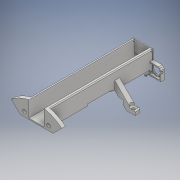
# Autodesk Inventor part: Hull_batt_pillar2
Saved by Autodesk Inventor 2018 (Build 220112000, 112)
## iProperties
Created: 2018-05-01
Part Number: Hull_batt_pillar2
Material: Generic
Document SubType Name: Modeling
Designer: suchanek
Density: 1 g/cm^3
Appearance: Default
Author: suchanek
Autodesk Inventor part; units mm, degrees
ref_plane "YZ Plane" through (0, 0, 0) normal (1, 0, 0) x (0, 1, 0)
ref_plane "XZ Plane" through (0, 0, 0) normal (0, 1, 0) x (-1, 0, 0)
ref_plane "XY Plane" through (0, 0, 0) normal (0, 0, 1) x (1, 0, 0)
sketch "Sketch1" plane through (0, 0, 0) normal (0, 1, 0) x (-1, 0, 0)
  arc A0 (21.0006, 25.4554) -> (6.35, 32.3833) centre (0, 0) ccw
  line L0 (0, 0) -> (-23.3345, 23.3345)
  line L1 (0, 0) -> (33, 0) construction
  line L2 (0, 0) -> (0, 8.3369)
  line L3 (-23.3345, 23.3345) -> (-9.1924, 9.1924)
  line L4 (-9.1924, 9.1924) -> (-6.965, 11.4198)
  line L5 (-6.965, 11.4198) -> (-13.7089, 18.1636)
  line L6 (-21.1071, 25.5619) -> (-23.3345, 23.3345)
  line L7 (23.3345, 23.3345) -> (9.1924, 9.1924)
  line L8 (9.1924, 9.1924) -> (6.965, 11.4198)
  line L9 (6.965, 11.4198) -> (13.7089, 18.1636)
  line L10 (21.1071, 25.5619) -> (23.3345, 23.3345)
  line L11 (-6.35, 32.3833) -> (6.35, 32.3833)
  line L12 (6.35, 32.3833) -> (6.35, 19.1636)
  line L13 (6.35, 19.1636) -> (-6.35, 19.1636)
  line L14 (-6.35, 19.1636) -> (-6.35, 32.3833)
  line L15 (13.7089, 18.1636) -> (-13.7089, 18.1636)
  line L16 (-13.7089, 18.1636) -> (-21.1071, 25.5619)
  arc A1 (-6.35, 32.3833) -> (-21.0006, 25.4554) centre (0, 0) ccw
  arc A2 (6.35, 32.3833) -> (-6.35, 32.3833) centre (0, 0) ccw
  line L17 (13.7089, 18.1636) -> (21.1071, 25.5619)
  point P0 (-6.35, 31.3636)
  dimension "d0" = 33
  dimension "d1" = 33
  dimension "d2" = 135
  dimension "d3" = 3.15
  dimension "d4" = 20
  dimension "d5" = 32
  dimension "d7" = 12.2
  dimension "d8" = 12.7
  dimension "d33" = 18.1636
  constraints: 36 end point, 7 point on circle, 6 point on line, 5 parallel, 4 symmetric about line, 3 centre point, 3 horizontal, 2 perpendicular, 1 coincident, 1 equal length, 1 vertical
  measures "d0" radius of A0
  measures "d1" distance of L0.start L0.end
  measures "d2" angle of L1 L0
  measures "d3" distance of L4.end L3.end
  measures "d4" distance between parallel lines of L6 L4
  measures "d5" distance of point (0, 0) point (-6.35, 31.364)
  measures "d7" distance of L13.end point (-6.35, 31.364)
  measures "d8" distance of L12.end L13.end
  measures "d33" distance from line of L0.start L15
extrude "Extrusion1" add sketch "Sketch1" along normal blind 3 contours L17 L15 L16 A1 L14 L13 L12 A0
sketch "Sketch2" plane through (0, 3, 0) normal (0, 1, 0) x (1, 0, 0)
  arc A0 (6.35, -32.3833) -> (21.0006, -25.4554) centre (0, 0) ccw projected
  line L0 (8.35, -31.9261) -> (8.35, -18.1636)
  line L1 (13.7089, -18.1636) -> (-13.7089, -18.1636) projected
  line L2 (-8.35, -18.1636) -> (-8.35, -31.9261)
  arc A1 (-21.0006, -25.4554) -> (-6.35, -32.3833) centre (0, 0) ccw projected
  line L3 (-6.35, -19.1636) -> (6.35, -19.1636) projected
  line L4 (6.35, -32.3833) -> (6.35, -19.1636)
  line L5 (6.35, -19.1636) -> (-6.35, -19.1636)
  line L6 (-6.35, -32.3833) -> (-6.35, -19.1636) projected
  line L7 (-6.35, -19.1636) -> (-6.35, -32.3833)
  dimension "d14" = 2
  constraints: 10 end point, 3 vertical, 2 perpendicular, 2 point on circle, 2 point on line, 1 horizontal alignment
  measures "d14" distance between parallel lines of L6 L2
extrude "Extrusion2" add sketch "Sketch2" along normal blind 85
ref_plane "Work Plane1" through (8.35, 3, 18.1636) normal (-0.7071068, 0, -0.7071068) x (0, 1, 0)
sketch "Sketch4" plane through (8.35, 3, 18.1636) normal (-0.7071068, 0, -0.7071068) x (0, 1, 0)
  circle A0 centre (49, 6.9393) radius 8
  line L0 (85, -9.7316) -> (85, 0) projected
  line L1 (-3, 3.7893) -> (0, 3.7893) projected
  line L2 (49, -1.0607) -> (31, -1.0607)
  line L3 (31, -1.0607) -> (31, 14.9393)
  line L4 (31, 14.9393) -> (49, 14.9393)
  line L5 (49, 14.9393) -> (49, -1.0607)
  point P0 (-3, 6.9393)
  dimension "d19" = 16
  dimension "d20" = 36
  dimension "d21" = 3.15
  dimension "d22" = 18
  dimension "d23" = 16
  constraints: 8 end point, 2 parallel, 2 point on circle, 1 centre point, 1 horizontal, 1 perpendicular
  measures "d19" diameter of A0
  measures "d20" distance from line of L0 A0.centre
  measures "d21" distance from line of L1 A0.centre
  measures "d22" distance of L3.end L4.end
  measures "d23" distance of L2.end L3.end
extrude "Extrusion3" cut sketch "Sketch4" along normal through all both and the other way through all
ref_plane "Work Plane3" through (0, 88, 18.1636) normal (-1, 0, 0) x (0, 0, 1)
mirror "Mirror1" about plane through (0, 88, 18.1636) normal (-1, 0, 0) of "Extrusion3"
sketch "Sketch5" plane through (0, 88, 0) normal (0, 1, 0) x (1, 0, 0)
  line L0 (8.35, -30.3833) -> (-8.35, -30.3833)
  line L1 (-8.35, -30.3833) -> (-8.35, -31.3833)
  line L2 (-8.35, -31.3833) -> (8.35, -31.3833)
  line L3 (8.35, -31.3833) -> (8.35, -30.3833)
  line L4 (8.35, -31.9261) -> (8.35, -18.1636) projected
  arc A0 (6.35, -32.3833) -> (21.0006, -25.4554) centre (0, 0) ccw projected
  dimension "d27" = 16.7
  dimension "d28" = 1
  dimension "d29" = 1
  constraints: 8 end point, 2 parallel, 1 collinear, 1 horizontal, 1 perpendicular
  measures "d27" distance of L2.end L1.end
  measures "d28" distance of L1.end L0.end
  measures "d29" distance from line of A0.start L2
extrude "Extrusion4" cut sketch "Sketch5" against normal blind 1.1
fillet "Fillet1" radius 0.5 4 edges at (7.35, 86.9, 31.3833) (-7.35, 86.9, 31.3833) (-7.35, 86.9, 30.3833) (7.35, 86.9, 30.3833)
sketch "Sketch6" plane through (13.7089, 0, 18.1636) normal (0, 0, -1) x (-1, 0, 0)
  line L0 (8.4589, 16) -> (18.9589, 16)
  line L1 (18.9589, 16) -> (18.9589, 54)
  line L2 (18.9589, 54) -> (8.4589, 54)
  line L3 (8.4589, 54) -> (8.4589, 16)
  line L4 (13.7089, 0) -> (13.7089, 8.6013)
  line L5 (5.3589, 88) -> (22.0589, 88) projected
  dimension "d36" = 10.5
  dimension "d37" = 38
  dimension "d38" = 34
  constraints: 10 end point, 2 parallel, 1 horizontal, 1 perpendicular, 1 vertical, 1 other
  measures "d36" distance of L1.end L2.end
  measures "d37" distance of L0.end L1.end
  measures "d38" distance between parallel lines of L5 L2
extrude "Extrusion5" [suppressed]
sketch "Náčrt7" plane through (0, 0, 0) normal (0, -1, 0) x (1, 0, 0)
  circle A0 centre (-10, 22) radius 1.55
  line L0 (0, 0) -> (0, 4.6263)
  circle A1 centre (10, 22) radius 1.55
  dimension "d39" = 22
  dimension "d40" = 10
  dimension "d41" = 3.1
  constraints: 2 centre point, 2 end point, 1 symmetric about line, 1 vertical, 1 other
  measures "d39" vertical distance of L0.start A0.centre
  measures "d40" horizontal distance of L0.start A0.centre
  measures "d41" diameter of A0
extrude "Vysunutí6" cut sketch "Náčrt7" against normal up to surface (3 mm away)
sketch "Náčrt8" plane through (0, 0, 0) normal (0, -1, 0) x (1, 0, 0)
  line L0 (-10, 19.1132) -> (-12.5, 20.5566)
  line L1 (-12.5, 20.5566) -> (-12.5, 23.4434)
  line L2 (-12.5, 23.4434) -> (-10, 24.8868)
  line L3 (-10, 24.8868) -> (-7.5, 23.4434)
  line L4 (-7.5, 23.4434) -> (-7.5, 20.5566)
  line L5 (-7.5, 20.5566) -> (-10, 19.1132)
  point P0 (0, 0)
  point P1 (-10, 22)
  point P2 (-10, 22)
  dimension "d44" = 2.5
  constraints: 12 end point, 1 coincident, 13 other
  measures "d44" distance from line of L4 point (-10, 22)
extrude "Vysunutí7" cut sketch "Náčrt8" against normal blind 2 from surface at -3
ref_plane "Pracovní rovina4" through (0, 0, 19.1636) normal (-1, 0, 0) x (0, 0, 1)
mirror "Zrcadlit2" about plane through (0, 0, 19.1636) normal (-1, 0, 0) of "Vysunutí7"
ref_plane "Pracovní rovina5" through (0, 60.8, 0) normal (0, 1, 0) x (1, 0, 0)
sketch "Náčrt12" plane through (0, 60.8, 0) normal (0, 1, 0) x (1, 0, 0)
  line L0 (8.35, 44.2663) -> (8.35, 40.3981)
  line L1 (8.35, 44.2663) -> (8.35, -18.1636)
  line L2 (18.1632, -8.3504) -> (25.2343, -8.3504)
  line L3 (21.8833, -11.7014) -> (8.35, -25.2347)
  line L4 (8.35, -18.1636) -> (8.35, -25.2347)
  line L5 (15.201, -14.8127) -> (15.201, -11.3127)
  line L6 (15.201, -14.8127) -> (11.701, -14.8127)
  line L7 (8.35, -18.1636) -> (11.701, -14.8127)
  line L8 (15.201, -11.3127) -> (18.1632, -8.3504)
  line L9 (25.2343, -8.3504) -> (25.2343, -10.7014)
  line L10 (24.2343, -11.7014) -> (21.8833, -11.7014)
  arc A0 (24.2343, -11.7014) -> (25.2343, -10.7014) centre (24.2343, -10.7014) ccw
  line L11 (8.35, -23.9341) -> (8.35, -20.0659) projected
  line L12 (8.35, -18.1636) -> (8.35, -20.0659) projected
  line L13 (8.35, -18.1636) -> (8.35, -19.6637) projected
  line L14 (8.35, -19.6637) -> (8.35, -18.1636) projected
  line L15 (8.35, -30.3833) -> (8.35, -18.1636) projected
  line L16 (8.35, -31.3833) -> (8.35, -30.3833) projected
  line L17 (8.35, -31.9261) -> (8.35, -31.3833) projected
  line L18 (8.35, -23.9341) -> (8.35, -31.9261) projected
  point P0 (0, 0)
  point P1 (25.3503, 46.1686)
  dimension "d72" = 13.878
  dimension "d73" = 1
  dimension "d74" = 3.5
  dimension "d75" = 5
  dimension "d76" = 3.351
  dimension "d77" = 16.8843
  dimension "d78" = 10.0333
  dimension "d79" = 45
  dimension "d80" = 90
  dimension "d81" = 135
  dimension "d82" = 135
  constraints: 22 end point, 3 collinear, 2 parallel, 2 perpendicular, 2 point on circle, 2 tangent, 1 centre point, 1 point on line
  measures "d72" distance of L1.end L2.start
  measures "d73" radius of A0
  measures "d74" distance of L5.start L6.end
  measures "d75" distance between parallel lines of L3 L8
  measures "d76" distance between parallel lines of L10 L2
  measures "d77" distance from line of L9 L0.start
  measures "d78" distance between parallel lines of L9 L5
  measures "d79" angle of L1 L3
  measures "d80" angle of L2 L9
  measures "d81" angle of L7 L6
  measures "d82" angle of L8 L5
extrude "Vysunutí11" add sketch "Náčrt12" against normal blind 4
sketch "Sketch15" plane through (21.8833, 60.8, 11.7014) normal (0, 0, 1) x (1, 0, 0)
  line L0 (0, 0) -> (0, -4) projected
  point P0 (-21.8833, -60.8)
  point P1 (0, -2)
  constraints: 1 midpoint
hole "Hole1" at (21.8833, 58.8, 11.7014) direction (0, 0, -1) diameter 2.5 end through all start extended yes countersink diameter 4.7 countersink angle 90
mirror "Mirror5" about plane through (0, 0, 19.1636) normal (-1, 0, 0) of "Vysunutí11", "Hole1"
sketch "Sketch16" plane through (0, 88, 0) normal (0, 1, 0) x (1, 0, 0)
  circle A0 centre (12.45, -19.1636) radius 4
  line L0 (17.45, -24.1636) -> (7.45, -24.1636)
  line L1 (7.45, -24.1636) -> (7.45, -14.1636)
  line L2 (7.45, -14.1636) -> (17.45, -14.1636)
  line L3 (17.45, -14.1636) -> (17.45, -24.1636)
  line L4 (-6.35, -19.1636) -> (6.35, -19.1636) projected
  line L5 (8.35, -30.3833) -> (8.35, -18.1636) projected
  point P0 (0, 0)
  dimension "d97" = 8
  dimension "d98" = 10
  dimension "d99" = 5
  dimension "d100" = 5
  dimension "d101" = 10
  dimension "d102" = 0.9
  constraints: 8 end point, 2 parallel, 1 centre point, 1 horizontal, 1 perpendicular, 1 point on line
  measures "d97" diameter of A0
  measures "d98" distance of L2.end L0.start
  measures "d99" distance from line of L3 A0.centre
  measures "d100" distance from line of L2 A0.centre
  measures "d101" distance of L1.end L2.end
  measures "d102" distance between parallel lines of L1 L5
extrude "Extrusion14" add sketch "Sketch16" along normal blind 1
sketch "Sketch17" plane through (0, 89, 0) normal (0, 1, 0) x (1, 0, 0)
  line L0 (7.45, -14.1636) -> (7.45, -24.1636) projected
  line L1 (17.45, -14.1636) -> (7.45, -14.1636) projected
  line L2 (7.45, -24.1636) -> (8.35, -24.1636)
  line L3 (8.35, -24.1636) -> (8.35, -14.1636)
  line L4 (8.35, -14.1636) -> (7.45, -14.1636)
  line L5 (7.45, -14.1636) -> (7.45, -24.1636)
  line L6 (17.45, -14.1636) -> (8.35, -14.1636)
  line L7 (8.35, -14.1636) -> (8.35, -15.0636)
  line L8 (8.35, -15.0636) -> (17.45, -15.0636)
  line L9 (17.45, -15.0636) -> (17.45, -14.1636)
  line L10 (7.45, -24.1636) -> (17.45, -24.1636) projected
  line L11 (17.45, -15.0636) -> (16.55, -15.0636)
  line L12 (16.55, -15.0636) -> (16.55, -24.1636)
  line L13 (16.55, -24.1636) -> (17.45, -24.1636)
  line L14 (17.45, -24.1636) -> (17.45, -15.0636)
  line L15 (8.35, -23.2636) -> (16.55, -23.2636)
  line L16 (16.55, -23.2636) -> (16.55, -24.1636)
  line L17 (16.55, -24.1636) -> (8.35, -24.1636)
  line L18 (8.35, -24.1636) -> (8.35, -23.2636)
  point P0 (0, 0)
  dimension "d105" = 0.9
  dimension "d107" = 0.9
  dimension "d108" = 0.9
  dimension "d111" = 0.9
  constraints: 32 end point, 8 parallel, 6 horizontal, 4 perpendicular, 3 point on line, 2 collinear, 2 other
  measures "d105" distance between parallel lines of L14 L12
  measures "d107" distance between parallel lines of L5 L3
  measures "d108" distance between parallel lines of L15 L17
  measures "d111" distance of L8.end L1.start
extrude "Extrusion15" add sketch "Sketch17" against normal blind 3 contours L1 L3 L2 L0 | L1 L9 L8 L3 | L3 L15 L12 L10 | L12 L8 L14 L10
sketch "Sketch18" plane through (17.45, 89, 24.1636) normal (1, 0, 0) x (0, 0, -1)
  line L0 (10, -3) -> (0, -3) projected
  line L1 (3, -3) -> (3.25, -3)
  line L2 (3.25, -3) -> (3.25, -1)
  line L3 (3.25, -1) -> (3, -1)
  line L4 (3, -1) -> (3, -3)
  line L5 (4.25, -3) -> (4.5, -3)
  line L6 (4.5, -3) -> (4.5, -1)
  line L7 (4.5, -1) -> (4.25, -1)
  line L8 (4.25, -1) -> (4.25, -3)
  line L9 (0, 0) -> (10, 0) projected
  line L10 (0, -3) -> (0, 0) projected
  point P0 (24.1636, -89)
  dimension "d112" = 1
  dimension "d113" = 0.25
  dimension "d114" = 0.25
  dimension "d115" = 1
  dimension "d116" = 3
  constraints: 16 end point, 4 parallel, 2 horizontal, 2 perpendicular, 2 point on line, 1 collinear
  measures "d112" distance between parallel lines of L9 L3
  measures "d113" distance between parallel lines of L4 L2
  measures "d114" distance of L6.end L7.end
  measures "d115" distance between parallel lines of L8 L2
  measures "d116" distance between parallel lines of L10 L4
extrude "Extrusion16" cut sketch "Sketch18" against normal blind 1
sketch "Sketch19" plane through (0, 86, 0) normal (0, -1, 0) x (1, 0, 0)
  line L0 (16.55, 20.9136) -> (16.55, 19.9136) projected
  line L1 (17.45, 19.9136) -> (17.45, 20.9136) projected
  line L2 (16.55, 20.9136) -> (17.45, 20.9136)
  line L3 (17.45, 20.9136) -> (17.45, 19.9136)
  line L4 (17.45, 19.9136) -> (16.55, 19.9136)
  line L5 (16.55, 19.9136) -> (16.55, 20.9136)
  point P0 (0, 0)
  constraints: 8 end point, 2 parallel, 1 horizontal, 1 perpendicular
extrude "Extrusion17" add sketch "Sketch19" along normal blind 3.5
sketch "Sketch20" plane through (16.55, 88, 19.9136) normal (-1, 0, 0) x (0, 0, 1)
  line L0 (1, -5.5) -> (1, 0) projected
  line L1 (1, -5.5) -> (0, -5.5)
  line L2 (0, -5.5) -> (0, -5)
  line L3 (0, -5) -> (1, -5)
  line L4 (1, -5) -> (1, -5.5)
  line L5 (0, 0) -> (0, -5.5) projected
  point P0 (-19.9136, -88)
  dimension "d121" = 0.5
  constraints: 8 end point, 2 parallel, 1 collinear, 1 horizontal, 1 perpendicular
  measures "d121" distance between parallel lines of L1 L3
extrude "Extrusion18" add sketch "Sketch20" along normal blind 0.5
chamfer "Chamfer1" distance 0.4 angle 45 1 edges at (16.05, 82.5, 20.4136)
sketch "Sketch21" plane through (8.35, 3, 31.9261) normal (1, 0, 0) x (0, 0, -1)
  line L0 (16.8625, 83) -> (13.7625, 83) projected
  line L1 (16.8625, 83) -> (16.6125, 83)
  line L2 (16.6125, 83) -> (16.6125, 85)
  line L3 (16.6125, 85) -> (16.8625, 85)
  line L4 (16.8625, 85) -> (16.8625, 83)
  line L5 (15.6125, 83) -> (15.3625, 83)
  line L6 (15.3625, 83) -> (15.3625, 85)
  line L7 (15.3625, 85) -> (15.6125, 85)
  line L8 (15.6125, 85) -> (15.6125, 83)
  line L9 (8.6625, 85) -> (16.8625, 85) projected
  point P0 (31.9261, -3)
  dimension "d127" = 1
  dimension "d128" = 0.25
  dimension "d129" = 0.25
  constraints: 16 end point, 4 parallel, 2 collinear, 2 horizontal, 2 perpendicular, 1 point on line
  measures "d127" distance between parallel lines of L8 L2
  measures "d128" distance between parallel lines of L4 L2
  measures "d129" distance between parallel lines of L8 L6
extrude "Extrusion19" cut sketch "Sketch21" against normal blind 1 contours L0 L2 L3 L4 | L0 L6 L7 L8
sketch "Sketch22" plane through (0, 86, 0) normal (0, -1, 0) x (1, 0, 0)
  line L0 (8.35, 15.3136) -> (8.35, 16.3136) projected
  line L1 (7.45, 16.3136) -> (7.45, 15.3136) projected
  line L2 (8.35, 16.3136) -> (7.45, 16.3136)
  line L3 (7.45, 16.3136) -> (7.45, 15.3136)
  line L4 (7.45, 15.3136) -> (8.35, 15.3136)
  line L5 (8.35, 15.3136) -> (8.35, 16.3136)
  point P0 (0, 0)
  constraints: 8 end point, 2 parallel, 1 horizontal, 1 perpendicular
extrude "Extrusion20" add sketch "Sketch22" along normal blind 3.5
sketch "Sketch23" plane through (8.35, 88, 16.3136) normal (1, 0, 0) x (0, 0, -1)
  line L0 (1, -5.5) -> (0, -5.5) projected
  line L1 (0, -5.5) -> (1, -5.5)
  line L2 (1, -5.5) -> (1, -5)
  line L3 (1, -5) -> (0, -5)
  line L4 (0, -5) -> (0, -5.5)
  line L5 (1, -5.5) -> (1, 0) projected
  point P0 (16.3136, -88)
  dimension "d134" = 0.5
  constraints: 8 end point, 2 parallel, 1 collinear, 1 horizontal, 1 perpendicular
  measures "d134" distance of L1.end L2.end
extrude "Extrusion21" add sketch "Sketch23" along normal blind 0.5
chamfer "Chamfer2" distance 0.4 angle 45 1 edges at (8.85, 82.5, 15.8136)
sketch "Sketch24" plane through (0, 88, 0) normal (0, 1, 0) x (1, 0, 0)
  line L0 (7.45, -18.1636) -> (-8.35, -18.1636) projected
  line L1 (7.45, -24.1636) -> (7.45, -18.1636) projected
  line L2 (-8.35, -18.1636) -> (7.45, -18.1636)
  line L3 (7.45, -18.1636) -> (7.45, -22.1636)
  line L4 (7.45, -22.1636) -> (-8.35, -22.1636)
  line L5 (-8.35, -22.1636) -> (-8.35, -18.1636)
  point P0 (0, 0)
  dimension "d140" = 4
  constraints: 8 end point, 2 parallel, 1 horizontal, 1 perpendicular, 1 point on line
  measures "d140" distance between parallel lines of L0 L4
extrude "Extrusion22" add sketch "Sketch24" along normal blind 0.25
sketch "Sketch25" plane through (0, 88.25, 0) normal (0, 1, 0) x (1, 0, 0)
  line L0 (7.45, -18.1636) -> (-8.35, -18.1636) projected
  line L1 (8.35, -31.9261) -> (8.35, -31.3833) projected
  line L2 (-8.35, -18.1636) -> (8.35, -18.1636)
  line L3 (8.35, -18.1636) -> (8.35, -31.9261)
  line L4 (8.35, -31.9261) -> (-8.35, -31.9261)
  line L5 (-8.35, -31.9261) -> (-8.35, -18.1636)
  point P0 (0, 0)
  constraints: 8 end point, 2 parallel, 1 horizontal, 1 perpendicular
extrude "Extrusion23" add sketch "Sketch25" along normal blind 0.75
sketch "Sketch26" plane through (0, 89, 0) normal (0, 1, 0) x (1, 0, 0)
  line L0 (7.3837, -32.3833) -> (21.5259, -18.2412)
  line L1 (6.8527, -32.3833) -> (26.8527, -32.3833) construction
  line L2 (21.5259, -18.2412) -> (21.5259, -32.3833)
  line L3 (21.5259, -32.3833) -> (7.3837, -32.3833)
  line L4 (8.35, -31.9261) -> (-8.35, -31.9261) projected
  point P0 (0, 0)
  point P1 (6.35, -32.3833)
  dimension "d145" = 45
  dimension "d146" = 20
  dimension "d150" = 0.36
  constraints: 8 end point, 2 point on line, 1 collinear, 1 equal length, 1 horizontal, 1 perpendicular
  measures "d145" angle of L1 L0
  measures "d146" distance of L0.start L0.end
  measures "d150" distance from line of L4.start L0
extrude "Extrusion24" cut sketch "Sketch26" against normal up to surface (86 mm away)
ref_plane "Work Plane6" through (0, 0, 32.3833) normal (1, 0, 0) x (0, 0, -1)
mirror "Mirror6" about plane through (0, 0, 32.3833) normal (1, 0, 0) of "Extrusion24"
sketch "Sketch29" plane through (-6.35, 0, 19.1636) normal (0, 0, 1) x (1, 0, 0)
  line L0 (8.5151, 45.35) -> (8.5151, 42.85)
  line L1 (8.5151, 42.85) -> (6.35, 41.6)
  line L2 (6.35, 41.6) -> (4.1849, 42.85)
  line L3 (4.1849, 42.85) -> (4.1849, 45.35)
  line L4 (4.1849, 45.35) -> (6.35, 46.6)
  line L5 (6.35, 46.6) -> (8.5151, 45.35)
  line L6 (12.7, 0) -> (12.7, 88) projected
  line L7 (0, 0) -> (12.7, 0) projected
  line L8 (-1.4909, 89) -> (14.1909, 89) projected
  point P0 (6.35, 0)
  point P1 (6.35, 44.1)
  point P2 (6.35, 0)
  dimension "d155" = 2.5
  dimension "d156" = 44.9
  constraints: 12 end point, 1 midpoint, 1 parallel, 1 vertical alignment, 13 other
  measures "d155" distance of L2.end L3.end
  measures "d156" distance from line of L8 point (6.35, 44.1)
extrude "Extrusion26" cut sketch "Sketch29" against normal through all
body "Solid1"
